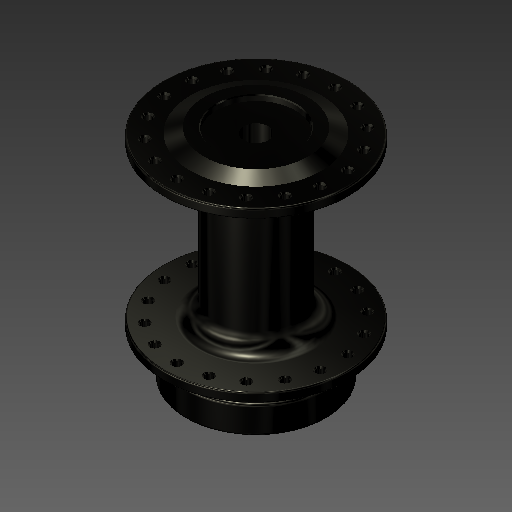
# Autodesk Inventor part: AmnzanaDel_68mm_disco
Saved by Autodesk Inventor 2018 (Build 220112000, 112)
## iProperties
Created: 2016-06-28
Part Number: AmnzanaDel_68mm_disco
Material: Aluminum 6061
Document SubType Name: Modeling
Designer: YeseF
Density: 2.7 g/cm^3
Appearance: Gunmetal
Author: YeseF
Autodesk Inventor part; units mm, degrees
ref_plane "YZ Plane" through (0, 0, 0) normal (1, 0, 0) x (0, 1, 0)
ref_plane "XZ Plane" through (0, 0, 0) normal (0, 1, 0) x (-1, 0, 0)
ref_plane "XY Plane" through (0, 0, 0) normal (0, 0, 1) x (1, 0, 0)
sketch "Sketch1" plane through (0, 0, 0) normal (0, 0, 1) x (1, 0, 0)
  line L0 (0, 0) -> (-15, 0)
  line L1 (-15, -27.5) -> (-15, 27.5)
  line L2 (0, -27.5) -> (0, 30.92)
  line L3 (0, -27.5) -> (-34, -27.5)
  line L4 (0, 27.5) -> (-34, 27.5)
  line L5 (0, -27.5) -> (0, -49)
  line L6 (0, -30.92) -> (-34, -30.92)
  line L7 (0, 30.92) -> (-34, 30.92)
  line L8 (0, -36.92) -> (-26, -36.92)
  line L9 (0, -47.08) -> (-26, -47.08)
  line L10 (-26, -47.08) -> (-26, -36.92)
  line L11 (-17.5, -36.92) -> (-17.5, -30.92)
  line L12 (-34, -30.92) -> (-34, -27.5)
  line L13 (-34, 27.5) -> (-34, 30.92)
  dimension "d3" = 15
  dimension "d4" = 55
  dimension "d5" = 34
  dimension "d6" = 34
  dimension "d7" = 21.5
  dimension "d8" = 3.42
  dimension "d9" = 3.42
  dimension "d10" = 6
  dimension "d11" = 26
  dimension "d12" = 19.58
  dimension "d13" = 17.5
  constraints: 28 end point, 8 point on line, 4 horizontal, 4 perpendicular, 3 vertical, 2 parallel, 1 midpoint
  measures "d3" distance of L0.end L0.start
  measures "d4" distance of L1.start L1.end
  measures "d5" distance of L2.start L3.end
  measures "d6" distance of L4.start L4.end
  measures "d7" distance of L2.start L5.end
  measures "d8" distance between parallel lines of L3 L6
  measures "d9" distance between parallel lines of L4 L7
  measures "d10" distance between parallel lines of L6 L8
  measures "d11" distance of L8.start L8.end
  measures "d12" distance between parallel lines of L3 L9
  measures "d13" distance between parallel lines of L5 L11
revolve "Revolution1" add sketch "Sketch1" angle 360 about axis through (0, -27.5, 0) along (0, 1, 0)
chamfer "Chamfer1" distance 10 angle 45 1 edges at (15, 27.5, 0)
fillet "Fillet1" radius 4 2 edges at (25, 27.5, 0) (15, 17.5, 0)
sketch "Sketch4" plane through (0, 30.92, 0) normal (0, 1, 0) x (1, 0, 0)
  line L0 (0, 0) -> (0, -29)
  circle A0 centre (0, -29) radius 1.35
  circle A1 centre (0, 0) radius 34 projected
  line L1 (0, -29) -> (0, -34)
  dimension "d19" = 2.7
  dimension "d21" = 5
  constraints: 4 end point, 2 vertical, 1 centre point, 1 coincident, 1 vertical alignment, 1 other
  measures "d19" diameter of A0
  measures "d21" distance of L1.start L1.end
extrude "Extrusion2" cut sketch "Sketch4" against normal through all contours A0 L1 L0 | L0 L1 A0
chamfer "Chamfer2" distance 0.5 angle 45 4 edges at (-1.35, 30.92, 29) (-1.35, 27.5, 29) (-1.35, -27.5, 29) (-1.35, -30.92, 29)
pattern_circular "Circular Pattern1" count 18 over 360 about axis through (0, 29.21, 0) along (0, 1, 0) of "Extrusion2", "Chamfer2"
sketch "Sketch5" plane through (0, -47.08, 0) normal (0, -1, 0) x (1, 0, 0)
  line L0 (0, 0) -> (0, 22)
  line L1 (0, 22) -> (0, 26)
  circle A0 centre (0, 22) radius 2.005
  circle A1 centre (0, 0) radius 26 projected
  dimension "d30" = 4.01
  dimension "d31" = 4
  constraints: 4 end point, 1 centre point, 1 coincident, 1 point on line, 1 vertical, 1 vertical alignment, 1 other
  measures "d30" diameter of A0
  measures "d31" distance of L0.end L1.end
extrude "Extrusion3" cut sketch "Sketch5" against normal up to surface (10.16 mm away) contours A0 L1 L0 | L0 L1 A0
chamfer "Chamfer3" distance 0.5 angle 45 2 edges at (-2.005, -47.08, 22) (-2.005, -36.92, 22)
pattern_circular "Circular Pattern2" count 6 over 360 about axis through (0, -42, 0) along (0, 1, 0) of "Extrusion3", "Chamfer3"
sketch "Sketch6" plane through (0, 30.92, 0) normal (0, 1, 0) x (1, 0, 0)
  circle A0 centre (0, 0) radius 19
  circle A1 centre (0, 0) radius 14.5
  dimension "d40" = 38
  dimension "d41" = 29
  constraints: 2 centre point, 2 coincident
  measures "d40" diameter of A0
  measures "d41" diameter of A1
extrude "Extrusion4" add sketch "Sketch6" along normal blind 2
chamfer "Chamfer4" distance 5 angle 21.8 1 edges at (-19, 30.92, 0) measured on face at (-23.2157, 30.92, -7.7273)
fillet "Fillet2" radius 6 1 edges at (15, -27.5, 0)
fillet "Fillet3" radius 2 2 edges at (17.5, -36.92, 0) (17.5, -30.92, 0)
fillet "Fillet4" radius 1 2 edges at (26, -36.92, 0) (26, -47.08, 0)
fillet "Fillet5" radius 0.6 4 edges at (34, -27.5, 0) (34, -30.92, 0) (34, 30.92, 0) (34, 27.5, 0)
sketch "Sketch7" plane through (0, -47.08, 0) normal (0, -1, 0) x (1, 0, 0)
  circle A0 centre (0, 0) radius 16.4
  circle A1 centre (0, 0) radius 14.5
  dimension "d51" = 32.8
  dimension "d52" = 29
  constraints: 2 centre point, 2 coincident
  measures "d51" diameter of A0
  measures "d52" diameter of A1
extrude "Extrusion5" add sketch "Sketch7" along normal blind 2
hole "Hole1" at (0, -47.08, 0) direction (0, 1, 0) diameter 9.02 end through all
chamfer "Chamfer5" distance 0.3 angle 45 3 edges at (-16.4, -49.08, 0) (-14.5, -49.08, 0) (-16.4, -47.08, 0)
chamfer "Chamfer6" distance 0.3 angle 45 1 edges at (-14.5, 32.92, 0)
equation "\"d6\" = d5"
equation "\"d9\" = d8"
body "Solid2"
